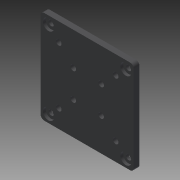
# Autodesk Inventor part: Topp 2.1
Saved by Autodesk Inventor 2015 (Build 190159000, 159)
## iProperties
Created: 2017-02-15
Part Number: Topp 2.1
Material: Generic
Document SubType Name: Modeling
Designer: Hampus
Density: 1 g/cm^3
Appearance: Gray
Author: Hampus
Autodesk Inventor part; units mm, degrees
ref_plane "YZ Plane" through (0, 0, 0) normal (1, 0, 0) x (0, 1, 0)
ref_plane "XZ Plane" through (0, 0, 0) normal (0, 1, 0) x (-1, 0, 0)
ref_plane "XY Plane" through (0, 0, 0) normal (0, 0, 1) x (1, 0, 0)
sketch "Sketch1" plane through (0, 0, 0) normal (0, 1, 0) x (-1, 0, 0)
  circle A0 centre (-17.5282, -17.6529) radius 1.5
  circle A1 centre (-32.4718, -17.6529) radius 1.5
  circle A2 centre (-32.4718, -32.3471) radius 1.5
  circle A3 centre (-40.25, -40.25) radius 1.5
  circle A4 centre (-40.25, -9.75) radius 1.5
  circle A5 centre (-17.5282, -32.3471) radius 1.5
  circle A6 centre (-9.75, -40.25) radius 1.5
  circle A7 centre (-9.75, -9.75) radius 1.5
  line L0 (0, 0) -> (0, -50)
  line L1 (0, -50) -> (-50, -50)
  line L2 (-50, -50) -> (-50, 0)
  line L3 (-50, 0) -> (0, 0)
  circle A8 centre (-4.2426, -4.2426) radius 1.5
  circle A9 centre (-4.2426, -45.7574) radius 1.5
  circle A10 centre (-45.7574, -45.7574) radius 1.5
  circle A11 centre (-45.7574, -4.2426) radius 1.5
  circle A12 centre (-6.6113, -80.0791) radius 3
  circle A13 centre (-15.9332, -80.0791) radius 3
  line L4 (-3.9183, -85.1543) -> (-3.9183, -133.5246) construction
  line L5 (-3.9183, -133.5246) -> (-20.8013, -133.5246) construction
  line L6 (-20.8013, -133.5246) -> (-20.8013, -85.1543) construction
  line L7 (-20.8013, -85.1543) -> (-3.9183, -85.1543) construction
  circle A14 centre (-4.2426, -4.2426) radius 3
  circle A15 centre (-4.2426, -45.7574) radius 3
  circle A16 centre (-45.7574, -45.7574) radius 3
  circle A17 centre (-45.7574, -4.2426) radius 3
  dimension "d2" = 3
  dimension "d3" = 3
  dimension "d4" = 3
  dimension "d5" = 3
  dimension "d6" = 50
  dimension "d7" = 50
  dimension "d12" = 3
  dimension "d13" = 3
  dimension "d14" = 3
  dimension "d15" = 3
  dimension "d16" = 6
  dimension "d17" = 6
  dimension "d21" = 6
  dimension "d22" = 6
  dimension "d23" = 6
  dimension "d24" = 6
  constraints: 18 centre point, 8 end point, 4 coincident, 2 parallel, 1 perpendicular, 2 other
  measures "d2" diameter of A7
  measures "d3" diameter of A4
  measures "d4" diameter of A3
  measures "d5" diameter of A6
  measures "d6" distance of L3.end L0.end
  measures "d7" distance of L3.start L3.end
  measures "d12" diameter of A8
  measures "d13" diameter of A9
  measures "d14" diameter of A10
  measures "d15" diameter of A11
  measures "d16" diameter of A13
  measures "d17" diameter of A12
  measures "d21" diameter of A14
  measures "d22" diameter of A15
  measures "d23" diameter of A16
  measures "d24" diameter of A17
extrude "Extrusion1" add sketch "Sketch1" along normal blind 3 contours L0 L1 L2 L3 | A14 | A15 | A16 | A17
fillet "Fillet1" radius 2 4 edges at (0, 1.5, -50) (50, 1.5, -50) (50, 1.5, 0) (0, 1.5, 0)
extrude "Extrusion2" cut sketch "Sketch1" along normal blind 1.5 contours A14 | A15 | A16 | A17
body "Solid1"
